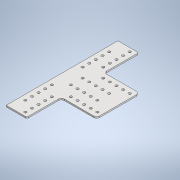
# Autodesk Inventor part: Lift.00.00.00.02
Saved by Autodesk Inventor 2021 (Build 250183000, 183)
## iProperties
Created: 2020-09-20
Part Number: Lift.00.00.00.02
Material: Типовые
Document SubType Name: ЛистМат
Designer: Kostya
Density: 1 g/cm^3
Appearance: По умолчанию
Sheet Metal Rule: По умолчанию_мм
Author: Kostya
Autodesk Inventor part; units mm, degrees
ref_plane "YZ Plane" through (0, 0, 0) normal (1, 0, 0) x (0, 1, 0)
ref_plane "XZ Plane" through (0, 0, 0) normal (0, 1, 0) x (-1, 0, 0)
ref_plane "XY Plane" through (0, 0, 0) normal (0, 0, 1) x (1, 0, 0)
sketch "Эскиз1" plane through (0, 0, 0) normal (0, 1, 0) x (-1, 0, 0)
  line L0 (0, 0) -> (386.4152, 0) construction
  line L1 (380, 0) -> (380, 380)
  line L2 (380, 380) -> (250, 380)
  line L3 (240, 370) -> (240, 165)
  line L4 (220, 145) -> (20, 145)
  line L5 (0, 125) -> (0, 0)
  circle A0 centre (275, 355) radius 8.5
  circle A1 centre (275, 310) radius 8.5
  circle A2 centre (275, 265) radius 8.5
  circle A3 centre (275, 220) radius 8.5
  circle A4 centre (275, 175) radius 8.5
  circle A5 centre (345, 285) radius 8.5
  circle A6 centre (345, 240) radius 8.5
  circle A7 centre (345, 195) radius 8.5
  circle A8 centre (345, 150) radius 8.5
  circle A9 centre (345, 105) radius 8.5
  circle A10 centre (30, 110) radius 8.5
  circle A11 centre (75, 110) radius 8.5
  circle A12 centre (120, 110) radius 8.5
  circle A13 centre (165, 110) radius 8.5
  circle A14 centre (210, 110) radius 8.5
  circle A15 centre (280, 40) radius 8.5
  circle A16 centre (235, 40) radius 8.5
  circle A17 centre (190, 40) radius 8.5
  circle A18 centre (145, 40) radius 8.5
  circle A19 centre (100, 40) radius 8.5
  arc A20 (20, 145) -> (0, 125) centre (20, 125) ccw
  arc A21 (250, 380) -> (240, 370) centre (250, 370) ccw
  arc A22 (220, 145) -> (240, 165) centre (220, 165) ccw
  line L6 (380, 0) -> (380, -380)
  line L7 (380, -380) -> (250, -380)
  line L8 (240, -370) -> (240, -165)
  line L9 (220, -145) -> (20, -145)
  line L10 (0, -125) -> (0, 0)
  circle A23 centre (275, -355) radius 8.5
  circle A24 centre (275, -310) radius 8.5
  circle A25 centre (275, -265) radius 8.5
  circle A26 centre (275, -220) radius 8.5
  circle A27 centre (275, -175) radius 8.5
  circle A28 centre (345, -285) radius 8.5
  circle A29 centre (345, -240) radius 8.5
  circle A30 centre (345, -195) radius 8.5
  circle A31 centre (345, -150) radius 8.5
  circle A32 centre (345, -105) radius 8.5
  circle A33 centre (30, -110) radius 8.5
  circle A34 centre (75, -110) radius 8.5
  circle A35 centre (120, -110) radius 8.5
  circle A36 centre (165, -110) radius 8.5
  circle A37 centre (210, -110) radius 8.5
  circle A38 centre (280, -40) radius 8.5
  circle A39 centre (235, -40) radius 8.5
  circle A40 centre (190, -40) radius 8.5
  circle A41 centre (145, -40) radius 8.5
  circle A42 centre (100, -40) radius 8.5
  arc A43 (0, -125) -> (20, -145) centre (20, -125) ccw
  arc A44 (240, -370) -> (250, -380) centre (250, -370) ccw
  arc A45 (240, -165) -> (220, -145) centre (220, -165) ccw
  point P0 (240, 380)
  point P1 (240, 145)
  point P2 (0, 145)
  point P3 (240, -380)
  point P4 (240, -145)
  point P5 (0, -145)
  dimension "d0" = 140
  dimension "d1" = 380
  dimension "d2" = 240
  dimension "d3" = 145
  dimension "d4" = 17
  dimension "d5" = 35
  dimension "d6" = 95
  dimension "d7" = 140
  dimension "d8" = 185
  dimension "d9" = 230
  dimension "d10" = 275
  dimension "d11" = 25
  dimension "d12" = 70
  dimension "d13" = 115
  dimension "d14" = 160
  dimension "d15" = 205
  dimension "d16" = 35
  dimension "d17" = 110
  dimension "d18" = 75
  dimension "d19" = 30
  dimension "d20" = 120
  dimension "d21" = 165
  dimension "d22" = 210
  dimension "d23" = 40
  dimension "d24" = 100
  dimension "d25" = 145
  dimension "d26" = 190
  dimension "d27" = 235
  dimension "d28" = 280
  dimension "d29" = 20
  dimension "d30" = 10
  measures "d0" distance of L1.end point (240, 380)
  measures "d1" distance between parallel lines of L2 L0
  measures "d2" distance of point (240, 145) point (0, 145)
  measures "d3" distance of point (0, 145) L0.start
  measures "d4" diameter of A0
  measures "d5" distance from line of A5.centre L1
  measures "d6" distance from line of L2 A5.centre
  measures "d7" distance from line of L2 A6.centre
  measures "d8" distance from line of L2 A7.centre
  measures "d9" distance from line of L2 A8.centre
  measures "d10" distance from line of L2 A9.centre
  measures "d11" distance from line of A0.centre L2
  measures "d12" distance from line of L2 A1.centre
  measures "d13" distance from line of L2 A2.centre
  measures "d14" distance from line of L2 A3.centre
  measures "d15" distance from line of L2 A4.centre
  measures "d16" distance from line of L3 A0.centre
  measures "d17" distance from line of L0 A10.centre
  measures "d18" distance from line of L5 A11.centre
  measures "d19" distance from line of L5 A10.centre
  measures "d20" distance from line of L5 A12.centre
  measures "d21" distance from line of L5 A13.centre
  measures "d22" distance from line of L5 A14.centre
  measures "d23" distance from line of L0 A19.centre
  measures "d24" distance from line of L5 A19.centre
  measures "d25" distance from line of L5 A18.centre
  measures "d26" distance from line of L5 A17.centre
  measures "d27" distance from line of L5 A16.centre
  measures "d28" distance from line of L5 A15.centre
  measures "d29" radius of A20
  measures "d30" radius of A21
extrude "Пластина1" add sketch "Эскиз1" along normal blind 10
equation "\"d31\" = Толщина"
equation "\"Глубина_просечки\" = 0.5 * Толщина"
equation "\"Толщина\" = 10"
